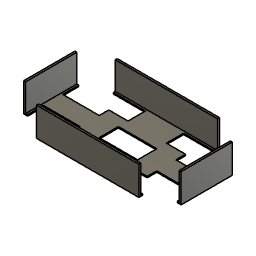
Grand guidage (Autodesk Fusion 360 design; units mm, degrees)
Autodesk Fusion 360 part; units mm, degrees
sketch "Esquisse1" plane through (0, 0, 0) normal (0, 1, 0) x (1, 0, 0)
  line L0 (0, 0) -> (160, 0)
  line L1 (160, 0) -> (160, -80)
  line L2 (160, -80) -> (0, -80)
  line L3 (0, -80) -> (0, 0)
  line L4 (-2, -30) -> (162, -30)
  line L5 (162, -30) -> (162, -50)
  line L6 (162, -50) -> (-2, -50)
  line L7 (-2, -50) -> (-2, -30)
  line L8 (60, 2) -> (100, 2)
  line L9 (100, 2) -> (100, -82)
  line L10 (100, -82) -> (60, -82)
  line L11 (60, -82) -> (60, 2)
  line L12 (-2, -40) -> (0, -40) construction
  line L13 (80, 0) -> (80, 2) construction
  line L14 (0, -40) -> (80, -40) construction
  line L15 (80, -40) -> (80, 0) construction
  line L16 (120, -20) -> (40, -20)
  line L17 (40, -20) -> (40, -60)
  line L18 (40, -60) -> (120, -60)
  line L19 (120, -60) -> (120, -20)
  line L20 (120, -20) -> (40, -60) construction
  line L21 (40, -20) -> (120, -60) construction
  line L22 (-2, -13.3333) -> (2, -13.3333)
  line L23 (2, -13.3333) -> (2, -66.6667)
  line L24 (2, -66.6667) -> (-2, -66.6667)
  line L25 (-2, -66.6667) -> (-2, -13.3333)
  line L26 (162, -66.6667) -> (158, -66.6667)
  line L27 (162, -13.3333) -> (162, -66.6667)
  line L28 (158, -66.6667) -> (158, -13.3333)
  line L29 (158, -13.3333) -> (162, -13.3333)
  line L30 (26.6667, -82) -> (133.3333, -82)
  line L31 (133.3333, -82) -> (133.3333, -78)
  line L32 (133.3333, -78) -> (26.6667, -78)
  line L33 (26.6667, -78) -> (26.6667, -82)
  line L34 (26.6667, -2) -> (133.3333, -2)
  line L35 (133.3333, -2) -> (133.3333, 2)
  line L36 (133.3333, 2) -> (26.6667, 2)
  line L37 (26.6667, 2) -> (26.6667, -2)
  point P0 (80, 0)
  point P1 (0, -40)
  point P2 (-2, -40)
  point P3 (80, 2)
  point P4 (80, -40)
  point P5 (80, -40)
  point P6 (-2, -40)
  point P7 (162, -40)
  point P8 (80, -82)
  point P9 (162, -40)
  dimension "d1" = 160
  dimension "d2" = 80
  dimension "d5" = 20
  dimension "d6" = 40
  dimension "d7" = 2
  dimension "d8" = 2
  dimension "d10" = 2
  dimension "d11" = 2
  dimension "d12" = 80
  dimension "d13" = 40
  dimension "d20" = 4
  dimension "d23" = 4
  dimension "d24" = 53.3333
  dimension "d25" = 53.3333
  dimension "d26" = 106.6667
  dimension "d27" = 106.6667
  dimension "d28" = 4
  dimension "d29" = 4
  constraint horizontal L0
  constraint vertical L1
  constraint horizontal L2
  constraint vertical L3
  constraint coincident L0.start L3.end
  constraint horizontal L4
  constraint vertical L5
  constraint horizontal L6
  constraint vertical L7
  constraint horizontal L8
  constraint vertical L9
  constraint horizontal L10
  constraint vertical L11
  constraint midpoint L0 P0
  constraint midpoint L3 P1
  constraint midpoint L8 P3
  constraint midpoint L7 P6
  constraint coincident P6 P2
  constraint coincident P1 L12.end
  constraint coincident P0 L13.start
  constraint coincident P3 L13.end
  constraint perpendicular L0 L13
  constraint perpendicular L3 L12
  constraint perpendicular L11 L14
  constraint perpendicular L0 L15
  constraint coincident P5 P4
  constraint horizontal L16
  constraint perpendicular L16 L17
  constraint parallel L16 L18
  constraint parallel L17 L19
  constraint coincident L20 P5
  constraint coincident L21 P5
  constraint horizontal L22
  constraint vertical L23
  constraint horizontal L24
  constraint vertical L25
  constraint midpoint L25 P6
  constraint midpoint P9 L27
  constraint midpoint L10 P8
  constraint midpoint L5 P9
  constraint perpendicular L27 L29
  constraint perpendicular L28 L29
  constraint perpendicular L26 L27
  constraint collinear L5 L27
  constraint horizontal L30
  constraint vertical L31
  constraint horizontal L32
  constraint vertical L33
  constraint midpoint P8 L30
  constraint horizontal L34
  constraint vertical L35
  constraint horizontal L36
  constraint vertical L37
  constraint midpoint P3 L36
  measures "d1" distance of L0.start L0.end
  measures "d2" distance of L0.start L2.end
  measures "d5" distance of L4.start L6.end
  measures "d6" distance of L8.start L8.end
  measures "d7" distance of L0 L8
  measures "d8" distance of L2 L10
  measures "d10" distance of L1 L5
  measures "d11" distance of L3 L7
  measures "d12" distance of L16.start L16.end
  measures "d13" distance of L16.start L18.end
  measures "d20" distance of L22.start L22.end
  measures "d23" distance of L26.start L26.end
  measures "d24" distance of L22.start L24.end
  measures "d25" distance of L26.start L27.start
  measures "d26" distance of L35.end L36.end
  measures "d27" distance of L30.start L30.end
  measures "d28" distance of L30.end L31.end
  measures "d29" distance of L34.end L35.end
extrude "Extrusion1" add sketch "Esquisse1" along normal blind 1.3 contours L0 L11 L34 L37 | L3 L4 L22 L23 | L0 L9 L11 L34 | L3 L4 L6 L23 | L0 L9 L34 L35 | L9 L11 L16 L34 | L3 L6 L23 L24 | L4 L6 L17 L23 | L4 L9 L11 L16 | L4 L11 L16 L17 | L4 L6 L11 L17 | L4 L9 L16 L19 | L6 L11 L17 L18 | L1 L4 L28 L29 | L4 L6 L9 L19 | L6 L9 L11 L18 | L2 L11 L32 L33 | L1 L4 L6 L28 | L4 L6 L19 L28 | L6 L9 L18 L19 | L9 L11 L18 L32 | L2 L9 L11 L32 | L1 L6 L26 L28 | L2 L9 L31 L32
extrude "Extrusion2" add sketch "Esquisse1" along normal blind 30 contours L0 L11 L36 L37 | L3 L4 L22 L25 | L0 L8 L9 L11 L36 | L3 L4 L6 L7 L25 | L0 L9 L35 L36 | L3 L6 L24 L25 | L1 L4 L27 L29 | L2 L11 L30 L33 | L1 L4 L5 L6 L27 | L2 L9 L10 L11 L30 | L1 L6 L26 L27 | L2 L9 L30 L31
equation "d1 = Longueur"
equation "d2 = Largeur"
equation "Longueur = 160 mm"
equation "Largeur = 80 mm"
equation "d5 = Largeur / 4"
equation "d6 = Longueur / 4"
equation "d7 = Epaisseur"
equation "d8 = Epaisseur"
equation "Epaisseur = 2 mm"
equation "d10 = Epaisseur"
equation "d11 = Epaisseur"
equation "d12 = Longueur / 2"
equation "d13 = Largeur / 2"
equation "d14 = hauteur_plaque"
equation "hauteur_plaque = 1.3 mm"
equation "hauteur_colonne = 30 mm"
equation "d18 = hauteur_colonne"
equation "d20 = Epaisseur * 2"
equation "d23 = Epaisseur * 2"
equation "d24 = Largeur / 1.5"
equation "d25 = Largeur / 1.5"
equation "d26 = Longueur / 1.5"
equation "d27 = Longueur / 1.5"
equation "d28 = Epaisseur * 2"
equation "d29 = Epaisseur * 2"
